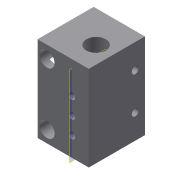
# Autodesk Inventor part: 30_CUBE_openXY_slider
Saved by Autodesk Inventor 2019 (Build 230136000, 136)
## iProperties
Created: 2020-01-07
Part Number: 30_CUBE_openXY_slider
Material: Generic
Document SubType Name: Modeling
Designer: diederichbenedict
Density: 1 g/cm^3
Appearance: Default
Author: diederichbenedict
Autodesk Inventor part; units mm, degrees
ref_plane "YZ Plane" through (0, 0, 0) normal (1, 0, 0) x (0, 1, 0)
ref_plane "XZ Plane" through (0, 0, 0) normal (0, 1, 0) x (-1, 0, 0)
sketch "Sketch1" plane through (0, 0, 0) normal (1, 0, 0) x (0, 1, 0)
  line L0 (0, 0) -> (35, 0)
  line L1 (35, 0) -> (35, 20)
  line L2 (35, 20) -> (0, 20)
  line L3 (0, 20) -> (0, 0)
  dimension "d0" = 35
  dimension "d1" = 20
  constraints: 8 end point, 2 parallel, 1 horizontal, 1 perpendicular
  measures "d0" distance of L2.end L1.end
  measures "d1" distance of L1.end L0.end
extrude "Extrusion1" add sketch "Sketch1" along normal blind 14
ref_plane "Work Plane1" through (7, 0, 0) normal (-1, 0, 0) x (0, 0, 1)
sketch "Sketch2" plane through (7, 0, 0) normal (-1, 0, 0) x (0, 0, 1)
  line L0 (20, 0) -> (0, 0) projected
  line L1 (10, 0) -> (10, 35)
  line L2 (0, 35) -> (20, 35) projected
  line L3 (3.8, 7.9) -> (16.2, 7.9)
  line L4 (16.2, 7.9) -> (16.2, 27.1)
  line L5 (16.2, 27.1) -> (3.8, 27.1)
  line L6 (3.8, 27.1) -> (3.8, 7.9)
  line L7 (3.8, 7.9) -> (16.2, 27.1) construction
  line L8 (16.2, 7.9) -> (3.8, 27.1) construction
  line L9 (10, 7.9) -> (6, 7.9)
  line L10 (6, 7.9) -> (6, 0)
  line L11 (6, 0) -> (10, 0)
  line L12 (10, 0) -> (10, 7.9)
  line L13 (10, 27.1) -> (6, 27.1)
  line L14 (6, 27.1) -> (6, 35)
  line L15 (6, 35) -> (10, 35)
  line L16 (10, 35) -> (10, 27.1)
  line L17 (10, 27.1) -> (3.8, 27.1)
  line L18 (3.8, 27.1) -> (3.8, 7.9)
  line L19 (3.8, 7.9) -> (10, 7.9)
  line L20 (10, 7.9) -> (10, 27.1)
  point P0 (10, 17.5)
  dimension "d5" = 12.4
  dimension "d6" = 19.2
  dimension "d7" = 4
  constraints: 38 end point, 8 parallel, 7 midpoint, 4 horizontal, 4 perpendicular, 3 point on line
  measures "d5" distance of L5.end L4.end
  measures "d6" distance of L4.end L3.end
  measures "d7" distance of L11.end L10.end
revolve "Revolution1" cut sketch "Sketch2" angle 360 about axis through (7, 0, 10) along (0, 1, 0) contours L0 L10 L3 L1 | L3 L6 L5 L1 | L5 L14 L2 L1
sketch "Sketch3" plane through (0, 0, 20) normal (0, 0, 1) x (1, 0, 0)
  line L0 (0, 35) -> (0, 0) projected
  line L1 (0, 0) -> (14, 0) projected
  line L2 (14, 35) -> (14, 0) projected
  line L3 (0, 35) -> (14, 35) projected
  line L4 (0, 0) -> (0, 35) projected
  line L5 (0, 0) -> (-7, 0)
  line L6 (-7, 0) -> (-7, 35)
  line L7 (-7, 35) -> (0, 35)
  line L8 (0, 35) -> (0, 0)
  line L9 (0, 35) -> (14, 35) projected
  circle A0 centre (-3.1, 5) radius 3.1
  line L10 (0, 35) -> (0, 0) projected
  circle A1 centre (-3.1, 30) radius 3.1
  dimension "d9" = 7
  dimension "d10" = 6.2
  dimension "d11" = 6.2
  dimension "d12" = 5
  dimension "d13" = 5
  constraints: 8 end point, 2 centre point, 2 parallel, 2 tangent, 1 horizontal, 1 perpendicular, 1 point on line
  measures "d9" distance of L6.end L7.end
  measures "d10" diameter of A0
  measures "d11" diameter of A1
  measures "d12" distance from line of A0.centre L5
  measures "d13" distance from line of A1.centre L7
extrude "Extrusion2" add sketch "Sketch3" against normal up to surface (20 mm away) contours L0 L5 L6 L7
sketch "Sketch4" plane through (-7, 0, 20) normal (-1, 0, 0) x (0, 0, 1)
  line L0 (-16.2, 27.1) -> (-16.2, 7.9) projected
  line L1 (-15, 24.5) -> (-5, 24.5) projected
  line L2 (-14, 27.1) -> (-6, 27.1) projected
  line L3 (-16.2, 7.9) -> (-3.8, 7.9) projected
  line L4 (-3.8, 27.1) -> (-3.8, 7.9) projected
  line L5 (-16.2, 27.1) -> (-3.8, 27.1) projected
  line L6 (-17, 27.5113) -> (-3, 27.5113)
  line L7 (-3, 27.5113) -> (-3, 7.5113)
  line L8 (-3, 7.5113) -> (-17, 7.5113)
  line L9 (-17, 7.5113) -> (-17, 27.5113)
  line L10 (-17, 27.5113) -> (-3, 7.5113) construction
  line L11 (-3, 27.5113) -> (-17, 7.5113) construction
  line L12 (-13.5, 32.7798) -> (-6.5, 32.7798)
  line L13 (-6.5, 32.7798) -> (-6.5, 27.5113)
  line L14 (-6.5, 27.5113) -> (-13.5, 27.5113)
  line L15 (-13.5, 27.5113) -> (-13.5, 32.7798)
  line L16 (-13.5, 32.7798) -> (-6.5, 27.5113) construction
  line L17 (-6.5, 32.7798) -> (-13.5, 27.5113) construction
  line L18 (-13.5, 1.8013) -> (-6.5, 1.8013)
  line L19 (-6.5, 1.8013) -> (-6.5, 7.5113)
  line L20 (-6.5, 7.5113) -> (-13.5, 7.5113)
  line L21 (-13.5, 7.5113) -> (-13.5, 1.8013)
  line L22 (-13.5, 1.8013) -> (-6.5, 7.5113) construction
  line L23 (-6.5, 1.8013) -> (-13.5, 7.5113) construction
  line L24 (0, 35) -> (-20, 35) projected
  line L25 (-13.5, 32.7798) -> (-6.5, 32.7798)
  line L26 (-6.5, 32.7798) -> (-6.5, 35)
  line L27 (-6.5, 35) -> (-13.5, 35)
  line L28 (-13.5, 35) -> (-13.5, 32.7798)
  line L29 (-6, 0) -> (-14, 0) projected
  line L30 (-13.5, 1.8013) -> (-6, 1.8013)
  line L31 (-6, 1.8013) -> (-6, 0)
  line L32 (-6, 0) -> (-13.5, 0)
  line L33 (-13.5, 0) -> (-13.5, 1.8013)
  point P0 (-20, 0)
  point P1 (-10, 17.5113)
  point P2 (-10, 30.1456)
  point P3 (-10, 4.6563)
  dimension "d16" = 14
  dimension "d17" = 20
  dimension "d18" = 7
  dimension "d41" = 7
  constraints: 52 end point, 10 parallel, 6 midpoint, 5 horizontal, 5 perpendicular, 4 point on line
  measures "d16" distance of L7.end L8.end
  measures "d17" distance of L6.end L7.end
  measures "d18" distance of L13.end L14.end
  measures "d41" distance between parallel lines of L19 L21
extrude "Extrusion3" cut sketch "Sketch4" against normal blind 12 contours L5 L2 L4 L3 L0 | L6 L7 L8 L9
sketch "Sketch5" plane through (14, 0, 0) normal (0, 0, -1) x (-1, 0, 0)
  line L0 (21, 35) -> (0, 35) projected
  line L1 (0, 0) -> (0, 35) projected
  line L2 (21, 0) -> (0, 0) projected
  line L3 (21, 35) -> (21, 0) projected
  circle A0 centre (17.1, 30) radius 3.1 projected
  circle A1 centre (17.1, 5) radius 3.1 projected
  point P0 (14, 0)
ref_plane "Work Plane2" through (-3.5, -134.0004, -5) normal (0, 0, -1) x (0, 1, 0)
extrude "Extrusion4" add sketch "Sketch5" along normal blind 3
sketch "Sketch6" plane through (-7, 0, 20) normal (-1, 0, 0) x (0, 0, 1)
  point P0 (-20, 0)
sketch "Sketch7" plane through (-7, 0, 20) normal (-1, 0, 0) x (0, 0, 1)
  line L0 (-3, 7.5113) -> (-17, 7.5113) projected
  line L1 (-17, 7.5113) -> (-17, 27.5113) projected
  line L2 (-17, 27.5113) -> (-3, 27.5113) projected
  line L3 (-3, 27.5113) -> (-3, 7.5113) projected
  line L4 (0, 0) -> (-23, 0) projected
  line L5 (0, 35) -> (0, 0) projected
  line L6 (0, 35) -> (-23, 35) projected
  line L7 (-23, 0) -> (-23, 35) projected
  circle A0 centre (-19, 10) radius 1.4
  circle A1 centre (-19, 25) radius 1.4
  point P0 (-20, 0)
  dimension "d23" = 2.8
  dimension "d24" = 2.8
  dimension "d25" = 10
  dimension "d26" = 10
  dimension "d27" = 4
  dimension "d36" = 4
  constraints: 2 centre point
  measures "d23" diameter of A0
  measures "d24" diameter of A1
  measures "d25" distance from line of A1.centre L6
  measures "d26" distance from line of L4 A0.centre
  measures "d27" distance from line of L7 A0.centre
  measures "d36" distance from line of L7 A1.centre
extrude "Extrusion5" cut sketch "Sketch7" against normal through all contours A0 | A1
sketch "Sketch8" plane through (14, 0, 20) normal (0, 0, 1) x (1, 0, 0)
  line L0 (-10, 99.8613) -> (-10, -100.1387)
  line L1 (-4, 99.8613) -> (-4, -100.1387)
  circle A0 centre (-7, 15) radius 1.4
  line L2 (-21, 0) -> (0, 0) projected
  circle A1 centre (-7, 8) radius 1.4
  circle A2 centre (-7, 22) radius 1.4
  point P0 (-14, 0)
  dimension "d31" = 2.8
  dimension "d32" = 15
  dimension "d33" = 3
  dimension "d37" = 2.8
  dimension "d38" = 2.8
  dimension "d39" = 7
  dimension "d40" = 7
  constraints: 4 end point, 3 centre point, 2 vertical, 4 other
  measures "d31" diameter of A0
  measures "d32" distance from line of L2 A0.centre
  measures "d33" distance from line of A0.centre L0
  measures "d37" diameter of A1
  measures "d38" diameter of A2
  measures "d39" distance of A0.centre A2.centre
  measures "d40" distance of A0.centre A1.centre
extrude "Extrusion6" cut sketch "Sketch8" against normal through all
body "Solid1"
